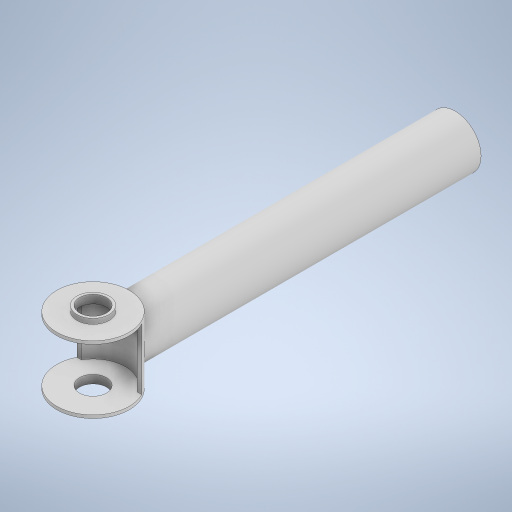
# Autodesk Inventor part: czlon_1
Saved by Autodesk Inventor 2023 (Build 270158000, 158)
## iProperties
Created: 2023-04-01
Part Number: czlon_1
Material: Ogólny
Document SubType Name: Modeling
Designer: krzys
Density: 1 g/cm^3
Appearance: Domyślna
Author: krzys
Autodesk Inventor part; units mm, degrees
ref_plane "YZ Plane" through (0, 0, 0) normal (1, 0, 0) x (0, 1, 0)
ref_plane "XZ Plane" through (0, 0, 0) normal (0, 1, 0) x (-1, 0, 0)
ref_plane "XY Plane" through (0, 0, 0) normal (0, 0, 1) x (1, 0, 0)
sketch "Szkic1" plane through (0, 0, 0) normal (0, 0, 1) x (1, 0, 0)
  circle A0 centre (0, 0) radius 50
  circle A1 centre (0, 0) radius 46
  circle A2 centre (0, 0) radius 31.5
  circle A3 centre (-28.9914, 28.9914) radius 4
  circle A4 centre (-28.9914, -28.9914) radius 4
  circle A5 centre (28.9914, 28.9914) radius 4
  circle A6 centre (28.9914, -28.9914) radius 4
  dimension "d0" = 100
  dimension "d1" = 92
  dimension "d2" = 63
  dimension "d4" = 8
  dimension "d5" = 8
  dimension "d6" = 8
  dimension "d7" = 8
  constraints: 7 centre point, 3 coincident
  measures "d0" diameter of A0
  measures "d1" diameter of A1
  measures "d2" diameter of A2
  measures "d4" diameter of A3
  measures "d5" diameter of A4
  measures "d6" diameter of A5
  measures "d7" diameter of A6
extrude "Wyciągnięcie proste1" add sketch "Szkic1" along normal blind 4 contours A1
extrude "Wyciągnięcie proste2" add sketch "Szkic1" along normal blind 700 contours A0
sketch "Szkic5" plane through (0, 0, 0) normal (0, 1, 0) x (-1, 0, 0)
  line L0 (50, 700) -> (-50, 700) projected
  circle A0 centre (0, 700) radius 70
  circle A1 centre (0, 700) radius 26
  circle A2 centre (0, 700) radius 62.5
  circle A3 centre (0, 700) radius 31
  line L1 (-62.5, 668.4762) -> (-53.9676, 668.4762)
  line L2 (53.9676, 668.4762) -> (62.5, 668.4762)
  point P0 (0, 0)
  point P1 (26, 700)
  point P2 (-26, 700)
  dimension "d28" = 140
  dimension "d29" = 52
  dimension "d34" = 125
  dimension "d35" = 62
  constraints: 4 centre point, 4 end point, 4 point on circle, 3 coincident, 1 midpoint
  measures "d28" diameter of A0
  measures "d29" diameter of A1
  measures "d34" diameter of A2
  measures "d35" diameter of A3
extrude "Wyciągnięcie proste7" add sketch "Szkic5" along normal mid plane 130 contours A3 L0 A1 | L0 A1 A3 | A1 L0 | L0 A1 | A0 L2 A2 L1 | L1 A2 L2 A0 | A2
extrude "Wyciągnięcie proste8" cut sketch "Szkic5" along normal mid plane 130 contours A1 L0 | L0 A1
extrude "Wyciągnięcie proste9" add sketch "Szkic5" along normal mid plane 150 contours A3 L0 A1 | L0 A1 A3
extrude "Wyciągnięcie proste10" cut sketch "Szkic5" along normal mid plane 118 contours A3 L0 A1 | L0 A1 A3 | A1 L0 | L0 A1 | A0 L2 A2 L1 | A2 picked at (-60.2574, 729.9527)
